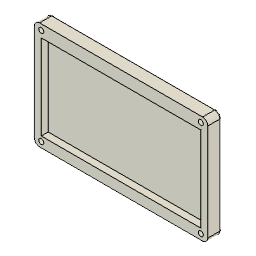
Alarm Clock Front (Autodesk Fusion 360 archive; units mm, degrees)
design "Alarm clock back"
part number: 2026-05-05-20-15-01-195
Autodesk Fusion 360 part; units mm, degrees
sketch "Sketch1" plane through (0, 0, 0) normal (0, 0, 1) x (1, 0, 0)
  line L0 (0, 0) -> (100, 0)
  line L1 (100, 0) -> (100, 62)
  line L2 (100, 62) -> (0, 62)
  line L3 (0, 62) -> (0, 0)
  line L4 (4, 55) -> (96, 55)
  line L5 (96, 55) -> (96, 6)
  line L6 (96, 6) -> (4, 6)
  line L7 (4, 6) -> (4, 55)
  dimension "d1" = 100
  dimension "d2" = 62
  dimension "d3" = 92
  dimension "d4" = 49
  dimension "d5" = 6
  dimension "d6" = 4
  constraint horizontal L0
  constraint vertical L1
  constraint horizontal L2
  constraint vertical L3
  constraint coincident L0.start L3.end
  constraint horizontal L4
  constraint vertical L5
  constraint horizontal L6
  constraint vertical L7
  measures "d1" distance of L0.start L0.end
  measures "d2" distance of L0.start L2.end
  measures "d3" distance of L4.start L4.end
  measures "d4" distance of L4.start L6.end
  measures "d5" distance of L0 L6
  measures "d6" distance of L3 L7
extrude "Extrude1" add sketch "Sketch1" along normal blind 2 contours L4 L5 L6 L7
extrude "Extrude2" add sketch "Sketch1" along normal blind 6
sketch "Sketch2" plane through (0, 0, 0) normal (0, 0, 1) x (1, 0, 0)
  line L0 (96, 52) -> (4, 52)
  line L1 (4, 52) -> (4, 10)
  line L2 (4, 10) -> (96, 10)
  line L3 (96, 10) -> (96, 52)
  line L4 (0, 0) -> (100, 0)
  line L5 (100, 0) -> (100, 62)
  dimension "d11" = 92
  dimension "d12" = 42
  dimension "d13" = 10
  dimension "d14" = 4
  constraint horizontal L0
  constraint vertical L1
  constraint horizontal L2
  constraint vertical L3
  measures "d11" distance of L0.start L0.end
  measures "d12" distance of L0.start L2.end
  measures "d13" distance of L2 L4
  measures "d14" distance of L3 L5
extrude "Extrude3" add sketch "Sketch1" against normal blind 2
ref_plane "WorkPlane1" through (0, 0, 15) normal (0, 0, 1) x (1, 0, 0)
sketch "Sketch3" plane through (0, 0, 15) normal (0, 0, 1) x (1, 0, 0)
  circle A0 centre (4, 3.25) radius 1.45
  circle A1 centre (96, 3.25) radius 1.45
  circle A2 centre (96, 58.75) radius 1.45
  circle A3 centre (4, 58.75) radius 1.45
  line L0 (0, 62) -> (0, 0)
  line L1 (0, 0) -> (100, 0)
  line L2 (100, 0) -> (100, 62)
  line L3 (100, 62) -> (0, 62)
  dimension "d18" = 2.9
  dimension "d19" = 2.9
  dimension "d20" = 2.9
  dimension "d21" = 2.9
  dimension "d22" = 4
  dimension "d23" = 3.25
  dimension "d24" = 4
  dimension "d25" = 3.25
  dimension "d26" = 4
  dimension "d27" = 3.25
  dimension "d28" = 4
  dimension "d29" = 3.25
  measures "d18" diameter of A0
  measures "d19" diameter of A1
  measures "d20" diameter of A2
  measures "d21" diameter of A3
  measures "d22" distance of A0.centre L0
  measures "d23" distance of A0.centre L1
  measures "d24" distance of A1.centre L2
  measures "d25" distance of A1.centre L1
  measures "d26" distance of A2.centre L2
  measures "d27" distance of A2.centre L3
  measures "d28" distance of A3.centre L0
  measures "d29" distance of A3.centre L3
extrude "Extrude4" cut sketch "Sketch3" against normal blind 25 contours A0 | A1 | A2 | A3
fillet "Fillet1" radius 3 4 edges at (100, 62, 2) (100, 0, 2) (0, 62, 2) (0, 0, 2)
fillet "Fillet2" radius 1 8 edges at (0.8787, 0.8787, -2) (0, 31, -2) (0.8787, 61.1213, -2) (50, 62, -2) (99.1213, 61.1213, -2) (100, 31, -2) (99.1213, 0.8787, -2) (50, 0, -2)
chamfer "Chamfer1" distance 1 angle 45 1 edges at (96, 30.5, -2)
chamfer "Chamfer2" distance 1 angle 45 1 edges at (4, 30.5, -2)
